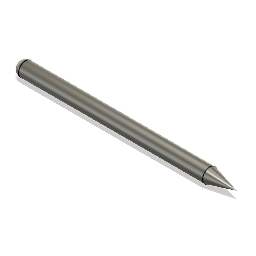
铅笔 (Autodesk Fusion 360 design; units mm, degrees)
Autodesk Fusion 360 part; units mm, degrees
sketch "草图2" plane through (0, 0, 0) normal (0, 1, 0) x (1, 0, 0)
sketch "草图3" plane through (0, 0, 0) normal (0, 1, 0) x (1, 0, 0)
sketch "草图4" plane through (0, 0, 0) normal (0, 0, 1) x (1, 0, 0)
cylinder "圆柱体基本要素2" add diameter 8 height 100 placed x (0, 0, -1) y (0, 1, 0) z (1, 0, 0) at (0, 30, 30) makes body 1
sphere "球体基本要素1" add diameter 8 placed x (1, 0, 0) y (0, 0, -1) z (0, 1, 0) at (15, 0, -25) separate body makes body 2
move_body "对齐1" bodies 2 to x (1, 0, 0) y (0, 1, 0) z (0, 0, 1) at (-15, 30, 55)
sketch "草图7" plane through (0, 0, 0) normal (0, 1, 0) x (1, 0, 0)
  line L0 (0, 10) -> (4, 10)
  line L1 (4, 10) -> (4, -5)
  line L2 (4, -5) -> (0, 10)
revolve "旋转1" add sketch "草图7" angle 360 about axis through (4, 0, -10) along (0, 0, 1) separate body makes body 3
move_body "对齐2" bodies 3 to x (0, 0, 1) y (0, -1, 0) z (1, 0, 0) at (110, 30, 26)
combine "合并1" operation add target body 3 tool bodies 1 2
